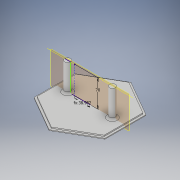
# Autodesk Inventor part: mounter
Saved by Autodesk Inventor 2019.3 (Build 233278000, 278)
## iProperties
Created: 2018-10-05
Part Number: mounter
Material: Generic
Document SubType Name: Modeling
Designer: HIVE
Density: 1 g/cm^3
Appearance: Default
Author: HIVE
Autodesk Inventor part; units mm, degrees
ref_plane "XZ Plane" through (0, 0, 0) normal (0, 1, 0) x (-1, 0, 0)
sketch "Sketch2" plane through (0, 0, 0) normal (0, 0, 1) x (1, 0, 0)
  line L0 (0, 0) -> (-38.9815, 0)
  line L1 (-46.3001, 0) -> (-38.9815, 0)
  line L2 (-38.9815, 0) -> (-31.6629, 0)
  line L3 (-49.7315, 70) -> (-64.9343, 70)
  line L4 (-64.9343, 70) -> (-64.9343, 0)
  line L5 (-64.9343, 0) -> (-49.7315, 0)
  line L6 (-49.7315, 0) -> (-49.7315, 70)
  line L7 (-38.9815, 70) -> (-38.9815, 0) construction
  line L8 (-57.3329, 70) -> (-57.3329, 0)
  dimension "d1" = 38.9815
  dimension "d53" = 70
  constraints: 19 end point, 3 collinear, 3 perpendicular, 2 horizontal, 2 midpoint, 1 coincident, 1 point on line, 1 vertical
  measures "d1" distance of L0.start L0.end
  measures "d53" distance of L7.start L0.end
sketch "Sketch3" plane through (0, 0, 0) normal (0, 1, 0) x (-1, 0, 0)
  circle A0 centre (0, 0) radius 105
  circle A1 centre (38.9815, 0) radius 7.3186 projected
  line L0 (0, -105) -> (-90.9327, -52.5)
  line L1 (-90.9327, -52.5) -> (-90.9327, 52.5)
  line L2 (-90.9327, 52.5) -> (0, 105)
  line L3 (0, 105) -> (90.9327, 52.5)
  line L4 (90.9327, 52.5) -> (90.9327, -52.5)
  line L5 (90.9327, -52.5) -> (0, -105)
  line L6 (-85.9327, -49.6132) -> (0, -99.2265)
  line L7 (0, -99.2265) -> (85.9327, -49.6132)
  line L8 (85.9327, -49.6132) -> (85.9327, 49.6132)
  line L9 (85.9327, 49.6132) -> (0, 99.2265)
  line L10 (0, 99.2265) -> (-85.9327, 49.6132)
  line L11 (-85.9327, 49.6132) -> (-85.9327, -49.6132)
  dimension "d14" = 210
  dimension "d15" = 5
  constraints: 24 end point, 2 coincident, 1 vertical, 1 vertical alignment, 20 other
  measures "d15" distance between parallel lines of L0 L6
extrude "Extrusion3" add sketch "Sketch3" against normal blind 5 contours A1 | L11 L10 L9 L8 L7 L6
extrude "Extrusion4" add sketch "Sketch3" along normal blind 2 from surface at -5 contours L4 L5 L0 L1 L2 L3
sketch "Sketch7" plane through (0, 0, 0) normal (0, 1, 0) x (-1, 0, 0)
  circle A0 centre (57.3329, 0) radius 7.6014
  line L0 (64.9343, 0) -> (49.7315, 0) projected
  point P0 (0, 0)
  point P1 (64.9343, 0)
  point P2 (64.9343, 0)
  point P3 (49.7315, 0)
  constraints: 2 point on circle, 1 centre point, 1 midpoint
sweep "Sweep1" add profiles "Sketch7" path "Sketch2" path curves L8
ref_plane "Work Plane1" through (-38.9815, 70, 0) normal (1, 0, 0) x (0, 1, 0)
sketch "Sketch8" plane through (-38.9815, 70, 0) normal (1, 0, 0) x (0, 1, 0)
  point P0 (-70, 0)
sketch "Sketch10" plane through (-38.9815, 70, 0) normal (1, 0, 0) x (0, 1, 0)
  line L0 (0, 0) -> (-25, 0) construction
  circle A0 centre (-25, 0) radius 5.5
  circle A1 centre (-25, 0) radius 9.5
  circle A2 centre (0, 0) radius 25 construction
  circle A3 centre (-19.2628, 15.9356) radius 9.5
  circle A4 centre (-19.2628, 15.9356) radius 5.5
  circle A5 centre (-4.6845, 24.5572) radius 9.5
  circle A6 centre (-4.6845, 24.5572) radius 5.5
  circle A7 centre (12.0438, 21.9077) radius 9.5
  circle A8 centre (12.0438, 21.9077) radius 5.5
  circle A9 centre (23.2444, 9.2031) radius 9.5
  circle A10 centre (23.2444, 9.2031) radius 5.5
  circle A11 centre (23.7764, -7.7254) radius 9.5
  circle A12 centre (23.7764, -7.7254) radius 5.5
  point P0 (-70, 0)
  dimension "d38" = 11
  dimension "d39" = 4
  dimension "d42" = 198
  dimension "d49" = 25
  constraints: 12 centre point, 2 coincident, 2 end point, 1 horizontal, 1 horizontal alignment, 18 other
  measures "d38" diameter of A0
  measures "d39" radial gap between concentric circles of A0 A1
  measures "d49" distance of L0.start L0.end
extrude "Extrusion9" [suppressed]
fillet "Fillet5" radius 5 1 edges at (-64.9343, 0, 0)
mirror "Mirror4" about plane through (0, 0, 0) normal (1, 0, 0) of "Sweep1", "Fillet5"
equation "\"d1\" = 0.5 * ballDist"
equation "\"ballDist\" = 77.963"
equation "\"ballDiam\" = 12.7"
equation "\"clearance\" = 0.4"
body "Solid1"
